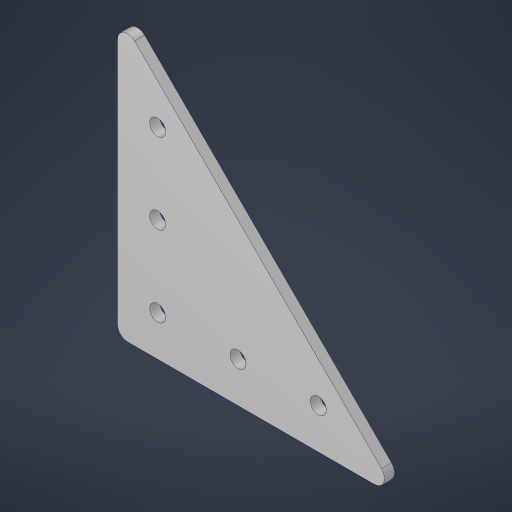
# Autodesk Inventor part: EL2-C-002
Saved by Autodesk Inventor 2023.4 (Build 274418000, 418)
## iProperties
Created: 2025-01-11
Part Number: EL2-C-002
Material: Aluminum 6061
Document SubType Name: Modeling
Designer: brand
Density: 2.7 g/cm^3
Appearance: Aluminum - Flat
Author: brand
Autodesk Inventor part; units mm, degrees
ref_plane "YZ Plane" through (0, 0, 0) normal (1, 0, 0) x (0, 1, 0)
ref_plane "XZ Plane" through (0, 0, 0) normal (0, 1, 0) x (-1, 0, 0)
ref_plane "XY Plane" through (0, 0, 0) normal (0, 0, 1) x (1, 0, 0)
sketch "Sketch1" plane through (0, 0, 0) normal (0, 0, 1) x (1, 0, 0)
  line L0 (0, 0) -> (88.9, 0)
  line L1 (0, 0) -> (0, 88.9)
  line L2 (0, 88.9) -> (88.9, 0)
  dimension "d0" = 88.9
  dimension "d1" = 88.9
  constraints: 6 end point, 1 horizontal, 1 vertical
  measures "d0" distance of L0.start L0.end
  measures "d1" distance of L0.start L1.end
extrude "Extrusion1" add sketch "Sketch1" along normal mid plane 3.175
fillet "Fillet1" radius 3.175 3 edges at (0, 88.9, 0) (88.9, 0, 0) (0, 0, 0)
sketch "Sketch2" plane through (0, 0, 1.5875) normal (0, 0, 1) x (1, 0, 0)
  arc A0 (0, 3.175) -> (3.175, 0) centre (3.175, 3.175) ccw construction
  line L0 (0, 3.175) -> (0, 81.2349) construction
  arc A1 (5.4201, 83.4799) -> (0, 81.2349) centre (3.175, 81.2349) ccw construction
  line L1 (5.4201, 83.4799) -> (83.4799, 5.4201) construction
  arc A2 (81.2349, 0) -> (83.4799, 5.4201) centre (81.2349, 3.175) ccw construction
  line L2 (81.2349, 0) -> (3.175, 0) construction
  point P0 (0, 0)
  point P1 (12.7, 12.7)
  dimension "d5" = 12.7
  dimension "d6" = 12.7
  measures "d5" distance from line of point (12.7, 12.7) L0
  measures "d6" distance from line of L2 point (12.7, 12.7)
hole "Hole1" at (12.7, 12.7, 1.5875) direction (0, 0, -1) diameter 5.1054 end through all clearance for "Flat Head Machine Screw (82)" size "#10" standard "Ansi Unified Screw Threads"
pattern_linear "Rectangular Pattern1" count 3 spacing 25.4 along (1, 0, 0) of "Hole1"
pattern_linear "Rectangular Pattern2" count 3 spacing 25.4 along (0, 1, 0) of "Hole1"
body "Solid1"
